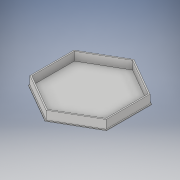
# Autodesk Inventor part: Screen2
Saved by Autodesk Inventor 2019 (Build 230136000, 136)
## iProperties
Created: 2020-07-28
Part Number: Screen2
Material: Genérico
Document SubType Name: Modeling
Designer: fga_d
Density: 1 g/cm^3
Appearance: Valor por defecto
Author: fga_d
Autodesk Inventor part; units mm, degrees
ref_plane "YZ Plane" through (0, 0, 0) normal (1, 0, 0) x (0, 1, 0)
ref_plane "XZ Plane" through (0, 0, 0) normal (0, 1, 0) x (-1, 0, 0)
ref_plane "XY Plane" through (0, 0, 0) normal (0, 0, 1) x (1, 0, 0)
sketch "Boceto2" plane through (0, 0, 0) normal (0, 1, 0) x (-1, 0, 0)
  line L0 (-73.6122, -42.5) -> (-73.6122, 127.5)
  line L1 (-73.6122, -42.5) -> (-147.2243, 0)
  line L2 (-147.2243, 0) -> (-147.2243, 85)
  line L3 (-147.2243, 85) -> (-73.6122, 127.5)
  line L4 (-73.6122, 127.5) -> (0, 85)
  line L5 (0, 85) -> (0, 0)
  line L6 (0, 0) -> (-73.6122, -42.5)
  point P0 (0, 0)
  point P1 (-60, 40)
  point P2 (-73.6122, 42.5)
  dimension "d1" = 170
  constraints: 14 end point, 1 vertical, 13 other
  measures "d1" distance of L0.start L0.end
extrude "Extrusión1" add sketch "Boceto2" along normal blind 1
sketch "Boceto3" plane through (0, 1, 0) normal (0, 1, 0) x (1, 0, 0)
  line L0 (147.2243, 0) -> (73.6122, 42.5) projected
  line L1 (73.6122, 42.5) -> (73.6122, -127.5)
  circle A0 centre (73.6122, -42.5) radius 82.95
  circle A1 centre (73.6122, -42.5) radius 80.3
  line L2 (73.6122, 40.45) -> (145.449, -1.025)
  line L3 (145.449, -1.025) -> (145.449, -83.975)
  line L4 (145.449, -83.975) -> (73.6122, -125.45)
  line L5 (73.6122, -125.45) -> (1.7754, -83.975)
  line L6 (1.7754, -83.975) -> (1.7754, -1.025)
  line L7 (1.7754, -1.025) -> (73.6122, 40.45)
  line L8 (73.6122, 37.8) -> (143.154, -2.35)
  line L9 (143.154, -2.35) -> (143.154, -82.65)
  line L10 (143.154, -82.65) -> (73.6122, -122.8)
  line L11 (73.6122, -122.8) -> (4.0703, -82.65)
  line L12 (4.0703, -82.65) -> (4.0703, -2.35)
  line L13 (4.0703, -2.35) -> (73.6122, 37.8)
  point P0 (0, 0)
  dimension "d4" = 165.9
  dimension "d5" = 160.6
  constraints: 26 end point, 3 coincident, 2 point on line, 2 vertical alignment, 1 midpoint, 1 vertical, 30 other
extrude "Extrusión2" add sketch "Boceto3" along normal blind 16 contours L3 A1 L2 | A1 L8 L2 | L3 A1 L9 | L2 A1 L1 | L1 A1 L7 | L4 A1 L3 | L13 A1 L7 | L7 A1 L6 | A1 L4 L10 | L5 A1 L1 | L1 A1 L4 | A1 L5 L11 | L12 A1 L6 | L6 A1 L5
